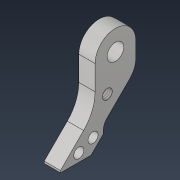
# Autodesk Inventor part: Chip Schaufel Seite
Saved by Autodesk Inventor 2022.3 (Build 263350000, 350)
## iProperties
Part Number: Chip Schaufel Seite
Material: Aluminium 6061
Document SubType Name: Modeling
Designer: rYan
Mass: 1.886 g
Surface Area: 7.62325 cm^2
Volume: 0.698518 cm^3
Density: 2.7 g/cm^3
Appearance: Aluminium - flach
Author: rYan
Autodesk Inventor part; units mm, degrees
ref_plane "YZ Plane" through (0, 0, 0) normal (1, 0, 0) x (0, 1, 0)
ref_plane "XZ Plane" through (0, 0, 0) normal (0, 1, 0) x (-1, 0, 0)
ref_plane "XY Plane" through (0, 0, 0) normal (0, 0, 1) x (1, 0, 0)
sketch "Skizze1" plane through (0, 0, 0) normal (1, 0, 0) x (0, 1, 0)
  line L0 (-4.8284, 6.1716) -> (-10.5, 0.5)
  line L1 (-10.5, 0) -> (-3, 0)
  line L2 (0, 3) -> (0, 5)
  line L3 (-10.5, 0.5) -> (-10.5, 0)
  line L4 (0, 5) -> (8, 13)
  circle A0 centre (3, 19) radius 0.5
  line L5 (-2, 13) -> (-2, 24)
  line L6 (-2, 24) -> (8, 24)
  line L7 (8, 24) -> (8, 13)
  line L8 (0, 3) -> (-3, 0)
  line L9 (8, 13) -> (-2, 13) construction
  line L10 (-4.8284, 6.1716) -> (8, 19) construction
  line L11 (0, 11) -> (5.3848, 24) construction
  line L12 (-15.5882, 0) -> (11.9314, 0) construction
  line L13 (3, 19) -> (3, 0) construction
  arc A1 (-4.8284, 6.1716) -> (-2, 13) centre (-11.6569, 13) ccw
  point P0 (0, 0)
  dimension "d67" = 0.5
  dimension "d69" = 1
  dimension "d72" = 10
  dimension "d73" = 45
  dimension "d76" = 45
  dimension "d91" = 19
  dimension "d92" = 3
  dimension "d93" = 5
  dimension "d96" = 10.5
  dimension "d97" = 0
  dimension "d98" = 3
  dimension "d99" = 5
  constraints: 27 end point, 6 point on line, 4 vertical, 3 perpendicular, 2 centre point, 2 point on circle, 2 tangent, 1 collinear, 1 horizontal, 1 parallel, 2 other
  measures "d67" distance of L0.end L3.end
  measures "d69" diameter of A0
  measures "d72" distance of L5.end L6.end
  measures "d73" angle of L8 L1
  measures "d76" angle of L0 L1
  measures "d91" vertical distance of point (0, 0) L13.start
  measures "d92" horizontal distance of point (0, 0) L13.start
  measures "d93" distance from line of L13.start L6
  measures "d96" distance from line of point (0, 0) L3
  measures "d97" distance from line of point (0, 0) L2
  measures "d98" distance of L1.end point (0, 0)
  measures "d99" distance of point (0, 0) L2.end
extrude "Extrusion1" add sketch "Skizze1" along normal mid plane 4
sketch "Skizze3" plane through (-2, 0, 0) normal (-1, 0, 0) x (0, 0, 1)
  line L0 (0, 11.7) -> (0, -14.2) projected
  circle A0 centre (19, 3) radius 0.5 projected
  constraints: 1 coincident
hole "Bohrung1" at (-2, 3, 19) direction (1, 0, 0) diameter 4.1 end through all
sketch "Skizze4" plane through (-2, 0, 0) normal (-1, 0, 0) x (0, 0, 1)
  line L0 (-4.8, 0) -> (28.8, 0) projected
  line L1 (0, 11.7) -> (0, -14.2) projected
  point P0 (11, 1)
  dimension "d37" = 11
  dimension "d95" = 1
  measures "d37" distance from line of L1 point (11, 1)
  measures "d95" distance from line of point (11, 1) L0
hole "Bohrung2" at (-2, 1, 11) direction (1, 0, 0) diameter 2.459 end through all thread size "M3x0.5" class "6H" standard "ISO Metric profile"
fillet "Rundung2" radius 5 3 edges at (0, 8, 24) (0, -2, 24) (0, 8, 13)
fillet "Rundung4" radius 3 3 edges at (0, -2, 13) (0, 0, 5) (0, -4.8284, 6.1716)
sketch "Skizze6" plane through (-2, 0, 0) normal (-1, 0, 0) x (0, 0, 1)
  line L0 (-4.8, 0) -> (28.8, 0) projected
  line L1 (0, 11.7) -> (0, -14.2) projected
  circle A0 centre (3.5, -2.5) radius 1.5 construction
  circle A1 centre (2, -6) radius 1.5 construction
  point P0 (0, 0)
  dimension "d80" = 3
  dimension "d81" = 3
  dimension "d87" = 1.5
  dimension "d88" = 3.5
  dimension "d89" = 2.5
  dimension "d90" = 3.5
  constraints: 2 centre point, 2 coincident
  measures "d80" diameter of A0
  measures "d81" diameter of A1
  measures "d87" horizontal distance of A1.centre A0.centre
  measures "d88" vertical distance of A1.centre A0.centre
  measures "d89" distance from line of A0.centre L0
  measures "d90" distance from line of L1 point (3.5, -2.5)
hole "Bohrung4" at (-2, -6, 2) at (-2, -2.5, 3.5) direction (1, 0, 0) diameter 2.5 end through all
